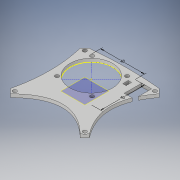
# Autodesk Inventor part: Fan_Mount
Saved by Autodesk Inventor 2019 (Build 230136000, 136)
## iProperties
Created: 2019-03-15
Part Number: Fan_Mount
Material: Generic
Document SubType Name: Modeling
Designer: Jorian Bruslind
Density: 1 g/cm^3
Appearance: Default
Author: Jorian Bruslind
Autodesk Inventor part; units mm, degrees
ref_plane "YZ Plane" through (0, 0, 0) normal (1, 0, 0) x (0, 1, 0)
ref_plane "XZ Plane" through (0, 0, 0) normal (0, 1, 0) x (-1, 0, 0)
ref_plane "XY Plane" through (0, 0, 0) normal (0, 0, 1) x (1, 0, 0)
sketch "Sketch1" plane through (0, 0, 0) normal (0, 1, 0) x (-1, 0, 0)
  circle A0 centre (0, 0) radius 48
  dimension "d0" = 96
  constraints: 1 centre point, 1 coincident
  measures "d0" diameter of A0
extrude "Extrusion1" add sketch "Sketch1" along normal blind 3
sketch "Sketch2" plane through (0, 3, 0) normal (0, 1, 0) x (1, 0, 0)
  circle A0 centre (-32, -32) radius 1.75
  line L0 (0, 0) -> (-48, 0)
  circle A1 centre (0, 0) radius 48 projected
  line L1 (0, 0) -> (0, -48)
  circle A2 centre (32, -32) radius 1.75
  circle A3 centre (32, 32) radius 1.75
  circle A4 centre (-32, 32) radius 1.75
  dimension "d3" = 3.5
  dimension "d4" = 32
  dimension "d5" = 32
  dimension "d8" = 360
  constraints: 4 centre point, 4 end point, 2 point on circle, 1 horizontal, 1 perpendicular, 9 other
  measures "d3" diameter of A0
  measures "d4" distance from line of L0 A0.centre
  measures "d5" distance from line of L1 A0.centre
extrude "Extrusion2" cut sketch "Sketch2" against normal blind 30 contours A0 | A2 | A3 | A4
sketch "Sketch3" plane through (0, 3, 0) normal (0, 1, 0) x (1, 0, 0)
  circle A0 centre (-32, 32) radius 1.75 projected
  line L0 (-30.25, 32) -> (-9.25, 32)
  circle A1 centre (0, 0) radius 48 projected
  line L1 (-9.25, 32) -> (-9.25, 15.135)
  line L2 (10.25, -4.365) -> (-28.75, 34.635) construction
  line L3 (-28.75, -4.365) -> (10.25, 34.635) construction
  circle A2 centre (-9.25, 15.135) radius 19.5
  dimension "d12" = 32
  dimension "d13" = 21
  dimension "d14" = 16.865
  dimension "d17" = 39
  constraints: 8 end point, 2 midpoint, 1 centre point, 1 coincident, 1 horizontal, 1 horizontal alignment, 1 vertical, 1 other
  measures "d12" distance from line of A1.centre L0
  measures "d13" distance of L0.start L0.end
  measures "d14" distance of L0.end L1.end
  measures "d17" diameter of A2
extrude "Extrusion3" cut sketch "Sketch3" against normal blind 5 contours A2
sketch "Sketch4" plane through (0, 0, 0) normal (0, -1, 0) x (1, 0, 0)
  line L0 (-29.25, 4.865) -> (10.75, 4.865)
  line L1 (10.75, 4.865) -> (10.75, -35.135)
  line L2 (10.75, -35.135) -> (-29.25, -35.135)
  line L3 (-29.25, -35.135) -> (-29.25, 4.865)
  circle A0 centre (-9.25, -15.135) radius 19.5 projected
  line L4 (-29.25, 4.865) -> (10.75, -35.135) construction
  line L5 (10.75, 4.865) -> (-29.25, -35.135) construction
  point P0 (0, 0)
  dimension "d20" = 40
  dimension "d21" = 40
  constraints: 12 end point, 2 midpoint, 2 parallel, 1 horizontal, 1 perpendicular
  measures "d20" distance of L1.end L2.end
  measures "d21" distance of L0.end L1.end
ref_plane "Work Plane1" through (0, 3, 0) normal (0, -1, 0) x (1, 0, 0)
sketch "Sketch5" plane through (0, 3, 0) normal (0, -1, 0) x (1, 0, 0)
  circle A0 centre (7.5, -31.135) radius 1.75
  line L0 (11.5, -35.135) -> (-28.5, -35.135) projected
  line L1 (11.5, 4.865) -> (11.5, -35.135) projected
  circle A1 centre (-8.5, -15.135) radius 19.5 projected
  circle A2 centre (-8.5, -15.135) radius 19.5
  circle A3 centre (7.5, 0.865) radius 1.75
  circle A4 centre (-24.5, 0.865) radius 1.75
  circle A5 centre (-24.5, -31.135) radius 1.75
  point P0 (0, 0)
  dimension "d24" = 3.5
  dimension "d25" = 4
  dimension "d26" = 4
  dimension "d27" = 39
  dimension "d30" = 360
  constraints: 5 centre point, 1 coincident, 9 other
  measures "d24" diameter of A0
  measures "d25" distance from line of L0 A0.centre
  measures "d26" distance from line of L1 A0.centre
  measures "d27" diameter of A2
extrude "Extrusion5" cut sketch "Sketch5" along normal blind 3 contours A0 | A3 | A4 | A5
sketch "Sketch7" plane through (0, 0, 0) normal (0, -1, 0) x (1, 0, 0)
  line L0 (0, 0) -> (0, 36)
  line L1 (0, 36) -> (-31.749, 36)
  circle A0 centre (0, 0) radius 48 projected
  line L2 (0, 36) -> (31.749, 36)
  line L3 (-28.5, 4.865) -> (11.5, 4.865) projected
  line L4 (31.749, 36) -> (0, 4.865) construction
  line L5 (0, 4.865) -> (-31.749, 36) construction
  spline S0 degree 2 poles (31.749, 36) (0, 4.865) (-31.749, 36) knots 1 1 1 2 2 2
  dimension "d52" = 36
  constraints: 6 end point, 3 point on line, 2 point on circle, 1 perpendicular, 1 vertical, 3 other
  measures "d52" distance of L0.start L0.end
extrude "Extrusion7" cut sketch "Sketch7" against normal blind 5 contours S0 L1 L0 | L0 L2 S0 | L1 A0 L2
sketch "Sketch8" plane through (0, 0, 0) normal (0, -1, 0) x (1, 0, 0)
  line L0 (0, 0) -> (36, 0)
  line L1 (36, 0) -> (36, -31.749)
  arc A0 (-31.749, 36) -> (31.749, 36) centre (0, 0) ccw projected
  line L2 (36, 0) -> (36, 31.749)
  line L3 (11.5, 4.865) -> (11.5, -35.135) projected
  line L4 (36, -31.749) -> (11.5, 0) construction
  line L5 (11.5, 0) -> (36, 31.749) construction
  spline S0 degree 2 poles (36, -31.749) (11.5, 0) (36, 31.749) knots 1 1 1 2 2 2
  dimension "d55" = 36
  constraints: 6 end point, 3 point on line, 2 point on circle, 1 horizontal, 1 vertical, 3 other
  measures "d55" distance of L0.start L0.end
extrude "Extrusion8" cut sketch "Sketch8" against normal blind 5
sketch "Sketch9" plane through (0, 0, 0) normal (0, -1, 0) x (1, 0, 0)
  line L0 (0, 0) -> (-36, 0)
  line L1 (-36, 0) -> (-36, 31.749)
  arc A0 (-31.749, 36) -> (36, -31.749) centre (0, 0) ccw projected
  line L2 (-36, 0) -> (-36, -31.749)
  line L3 (-28.5, -35.135) -> (-28.5, 4.865) projected
  line L4 (-36, 31.749) -> (-28.5, 0) construction
  line L5 (-28.5, 0) -> (-36, -31.749) construction
  spline S0 degree 2 poles (-36, 31.749) (-28.5, 0) (-36, -31.749) knots 1 1 1 2 2 2
  dimension "d58" = 36
  constraints: 6 end point, 3 point on line, 2 point on circle, 1 horizontal, 1 perpendicular, 3 other
  measures "d58" distance of L0.start L0.end
extrude "Extrusion9" cut sketch "Sketch9" against normal blind 5
sketch "Sketch10" plane through (0, 0, 0) normal (0, -1, 0) x (1, 0, 0)
  line L0 (0, 0) -> (0, -36)
  line L1 (0, -36) -> (-31.749, -36)
  line L2 (0, -36) -> (31.749, -36)
  line L3 (11.5, 4.865) -> (11.5, -35.135) projected
  arc A0 (-36, -31.749) -> (36, -31.749) centre (0, 0) ccw projected
  line L4 (-28.5, -36) -> (-28.5, -38.6232)
  line L5 (-28.5, -35.135) -> (-28.5, 4.865) projected
  line L6 (0, -36) -> (0, -39)
  line L7 (31.749, -36) -> (0, -39) construction
  line L8 (0, -39) -> (-28.5, -36) construction
  spline S0 degree 2 poles (31.749, -36) (0, -39) (-28.5, -36) knots 1 1 1 2 2 2
  arc A1 (-31.749, -36) -> (31.749, -36) centre (0, 0) ccw
  dimension "d61" = 36
  dimension "d69" = 31.749
  dimension "d71" = 2.6232
  dimension "d72" = 3
  constraints: 10 end point, 3 point on circle, 2 coincident, 2 point on line, 2 vertical, 1 centre point, 1 collinear, 1 horizontal, 3 other
  measures "d61" distance of L0.start L0.end
  measures "d69" distance of L0.end L2.end
  measures "d71" distance of L4.start L4.end
  measures "d72" distance of L0.end L6.end
sketch "Sketch11" plane through (0, 0, 0) normal (0, -1, 0) x (1, 0, 0)
  line L0 (11.5, 4.865) -> (11.5, -35.135) projected
  line L1 (11.5, -35.135) -> (11.5, -28.135)
  line L2 (11.5, -28.135) -> (14.5, -28.135)
  line L3 (14.5, -28.135) -> (14.5, -23.135)
  line L4 (14.5, -23.135) -> (11.5, -23.135)
  line L5 (11.5, -23.135) -> (11.5, -28.135)
  point P0 (0, 0)
  dimension "d64" = 7
  dimension "d65" = 3
  dimension "d66" = 5
  constraints: 10 end point, 2 parallel, 1 horizontal, 1 perpendicular, 1 point on line
  measures "d64" distance of L0.end L1.end
  measures "d65" distance of L4.end L3.end
  measures "d66" distance of L3.end L2.end
extrude "Extrusion11" cut sketch "Sketch11" against normal blind 5
extrude "Extrusion12" cut sketch "Sketch10" against normal blind 5 contours L4 A0 L1 | S0 A0 L4
sketch "Sketch13" plane through (0, 0, 0) normal (0, -1, 0) x (1, 0, 0)
  circle A0 centre (32, -32) radius 1.75 projected
  line L0 (32, -32) -> (28.23, -32)
  line L1 (28.23, -32) -> (28.23, -24.2)
  line L2 (28.23, -24.2) -> (24.23, -24.2)
  line L3 (19.73, -16.2) -> (28.73, -16.2)
  line L4 (28.73, -16.2) -> (28.73, -32.2)
  line L5 (28.73, -32.2) -> (19.73, -32.2)
  line L6 (19.73, -32.2) -> (19.73, -16.2)
  line L7 (19.73, -16.2) -> (28.73, -32.2) construction
  line L8 (28.73, -16.2) -> (19.73, -32.2) construction
  point P0 (0, 0)
  dimension "d82" = 3.77
  dimension "d83" = 7.8
  dimension "d84" = 4
  dimension "d85" = 9
  dimension "d86" = 16
  constraints: 18 end point, 3 perpendicular, 2 horizontal, 2 midpoint, 2 parallel
  measures "d82" distance of L0.start L0.end
  measures "d83" distance of L0.end L1.end
  measures "d84" distance of L1.end L2.end
  measures "d85" distance of L4.end L5.end
  measures "d86" distance of L3.end L4.end
extrude "Extrusion14" cut sketch "Sketch13" against normal blind 3 contours L3 L4 L5 L6
body "Solid1"
